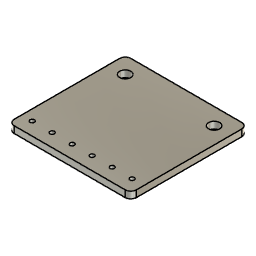
maze solevr part-1 v51 (Autodesk Fusion 360 archive; units mm, degrees)
design "ToF Distance Ranging Sensor"
Autodesk Fusion 360 part; units mm, degrees
sketch "Sketch1" plane through (0, 0, 0) normal (0, 0, 1) x (1, 0, 0)
  line L0 (21, 0.5) -> (21, 19.5)
  line L1 (-1, 19.5) -> (-1, 0.5)
  line L2 (20, 20.5) -> (0, 20.5)
  line L3 (0, -0.5) -> (20, -0.5)
  circle A0 centre (0.8946, 1.8577) radius 0.4
  circle A1 centre (4.4946, 1.8577) radius 0.4
  circle A2 centre (8.0946, 1.8577) radius 0.4
  circle A3 centre (11.6946, 1.8577) radius 0.4
  circle A4 centre (15.2946, 1.8577) radius 0.4
  circle A5 centre (18.8946, 1.8577) radius 0.4
  arc A6 (0, 20.5) -> (-1, 19.5) centre (0, 19.5) ccw
  arc A7 (21, 19.5) -> (20, 20.5) centre (20, 19.5) ccw
  arc A8 (-1, 0.5) -> (0, -0.5) centre (0, 0.5) ccw
  arc A9 (20, -0.5) -> (21, 0.5) centre (20, 0.5) ccw
  line L4 (-1, 20) -> (-1, 17.5)
  circle A10 centre (2, 17.5) radius 1
  circle A11 centre (18, 17.5) radius 1
  line L5 (17, 17.5) -> (18, 17.5)
  point P0 (20, 0)
  point P1 (0, 20)
  point P2 (9.789, 1.7034)
  point P3 (18.289, 1.7034)
  dimension "d1" = 20
  dimension "d2" = 20
  dimension "d30" = 0.8
  dimension "d33" = 18
  dimension "d34" = 0
  dimension "d35" = 1
  dimension "d36" = 2.5
  dimension "d37" = 3
  dimension "d38" = 2
  dimension "d39" = 2
  constraint tangent L2 A6
  constraint tangent L1 A6
  constraint tangent L2 A7
  constraint tangent L0 A7
  constraint equal A6 A7
  constraint tangent L1 A8
  constraint tangent L3 A8
  constraint equal A6 A8
  constraint tangent L0 A9
  constraint tangent L3 A9
  constraint equal A6 A9
  constraint parallel L1 L4
  constraint coincident A11.centre L5.end
  constraint coincident A11 L5.start
  measures "d1" distance of origin P0
  measures "d2" distance of origin P1
  measures "d30" diameter of A0
  measures "d35" radius of A6
  measures "d36" distance of L4.start L4.end
  measures "d37" distance of L4.end A10.centre
  measures "d38" diameter of A10
  measures "d39" diameter of A11
sketch "Sketch2" plane through (0, 0, 0) normal (0, 0, 1) x (1, 0, 0)
extrude "Extrude3" add sketch "Sketch1" along normal blind 1.21
extrude "Extrude2" [rolled back] along distance 1.21 taper angle 0

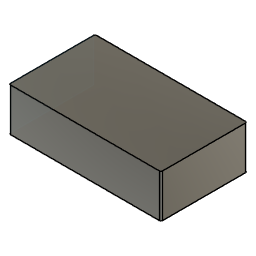
design "BATTERY"
Autodesk Fusion 360 part; units mm, degrees
sketch "Sketch1" plane through (0, 0, 0) normal (0, 0, 1) x (1, 0, 0)
  line L0 (0, 0) -> (53, 0)
  line L1 (53, 0) -> (53, 30)
  line L2 (53, 30) -> (0, 30)
  line L3 (0, 30) -> (0, 0)
  dimension "d1" = 53
  dimension "d2" = 30
  constraint horizontal L0
  constraint vertical L1
  constraint horizontal L2
  constraint vertical L3
  constraint coincident L0.start L3.end
  measures "d1" distance of L0.start L0.end
  measures "d2" distance of L0.start L2.end
extrude "Extrude1" add sketch "Sketch1" along normal blind 15
fillet "Fillet1" radius 0.5 1 edges at (0, 0, 7.5)
fillet "Fillet2" radius 0.5 3 edges at (53, 30, 7.5) (53, 0, 7.5) (0, 30, 7.5)
sketch "Sketch2" plane through (0, 0, 0) normal (-1, 0, 0) x (0, -1, 0)
  line L0 (-29.5, 15) -> (-29.5, 0)
  line L1 (-29.5, 0) -> (-0.5, 0)
  line L2 (-0.5, 0) -> (-0.5, 15)
  line L3 (-0.5, 15) -> (-29.5, 15)

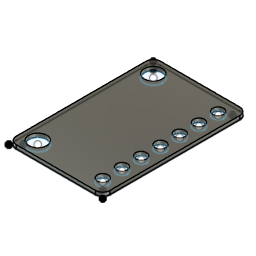
design "MAZE SOLVER WITH IMPELLER"
Autodesk Fusion 360 part; units mm, degrees
sketch "Sketch1" plane through (0, 0, 0) normal (0, 0, 1) x (1, 0, 0)
  line L0 (1, 0) -> (12, 0)
  line L1 (13, 1) -> (13, 19)
  line L2 (12, 20) -> (1, 20)
  line L3 (0, 19) -> (0, 1)
  circle A0 centre (2, 18) radius 1.25
  circle A1 centre (2, 2) radius 1.25
  arc A2 (1, 20) -> (0, 19) centre (1, 19) ccw
  arc A3 (0, 1) -> (1, 0) centre (1, 1) ccw
  arc A4 (13, 19) -> (12, 20) centre (12, 19) ccw
  arc A5 (12, 0) -> (13, 1) centre (12, 1) ccw
  circle A6 centre (11, 18) radius 0.75
  circle A7 centre (11, 15.3333) radius 0.75
  circle A8 centre (11, 12.6667) radius 0.75
  circle A9 centre (11, 10) radius 0.75
  circle A10 centre (11, 7.3333) radius 0.75
  circle A11 centre (11, 4.6667) radius 0.75
  circle A12 centre (11, 2) radius 0.75
  point P0 (13, 0)
  point P1 (0, 20)
  dimension "d1" = 13
  dimension "d2" = 20
  dimension "d3" = 2.5
  dimension "d4" = 2.5
  dimension "d5" = 1
  dimension "d6" = 1.5
  dimension "d9" = 0
  dimension "d10" = -16
  constraint horizontal L0
  constraint vertical L1
  constraint horizontal L2
  constraint vertical L3
  constraint coincident P1 L2
  constraint coincident P1 L3
  constraint tangent L2 A2
  constraint tangent L3 A2
  constraint coincident origin L3
  constraint coincident origin L0
  constraint tangent L3 A3
  constraint tangent L0 A3
  constraint equal A2 A3
  constraint tangent L2 A4
  constraint tangent L1 A4
  constraint equal A2 A4
  constraint coincident P0 L1
  constraint coincident P0 L0
  constraint tangent L1 A5
  constraint tangent L0 A5
  constraint equal A2 A5
  measures "d1" distance of origin P0
  measures "d2" distance of origin P1
  measures "d3" diameter of A0
  measures "d4" diameter of A1
  measures "d5" radius of A2
  measures "d6" diameter of A6
sketch "Sketch2" plane through (0, 0, 0) normal (0, 0, 1) x (1, 0, 0)
extrude "Extrude1" add sketch "Sketch1" along normal blind 0.5

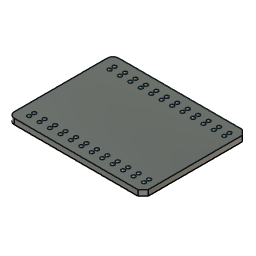
design "part-1 maze solver"
Autodesk Fusion 360 part; units mm, degrees
sketch "Sketch7" plane through (0, 0, 0) normal (0, 0, 1) x (1, 0, 0)
  line L0 (1.5, 0) -> (34.91, 0)
  line L1 (34.91, 28.14) -> (1.5, 28.14)
  line L2 (0, 26.64) -> (0, 1.5)
  line L3 (34.91, 28.14) -> (36.28, 26.77)
  line L4 (34.91, 0) -> (36.28, 1.37)
  arc A0 (1.5, 28.14) -> (0, 26.64) centre (1.5, 26.64) ccw
  arc A1 (0, 1.5) -> (1.5, 0) centre (1.5, 1.5) ccw
  circle A2 centre (3, 25.6) radius 0.5
  circle A3 centre (3, 24.23) radius 0.5
  circle A4 centre (3, 3.91) radius 0.5
  circle A5 centre (3, 2.54) radius 0.5
  circle A6 centre (5.8182, 25.6) radius 0.5
  circle A7 centre (5.8182, 24.23) radius 0.5
  circle A8 centre (8.6364, 25.6) radius 0.5
  circle A9 centre (8.6364, 24.23) radius 0.5
  circle A10 centre (11.4545, 25.6) radius 0.5
  circle A11 centre (11.4545, 24.23) radius 0.5
  circle A12 centre (14.2727, 24.23) radius 0.5
  circle A13 centre (17.0909, 25.6) radius 0.5
  circle A14 centre (17.0909, 24.23) radius 0.5
  circle A15 centre (19.9091, 25.6) radius 0.5
  circle A16 centre (19.9091, 24.23) radius 0.5
  circle A17 centre (22.7273, 25.6) radius 0.5
  circle A18 centre (22.7273, 24.23) radius 0.5
  circle A19 centre (25.5455, 25.6) radius 0.5
  circle A20 centre (25.5455, 24.23) radius 0.5
  circle A21 centre (28.3636, 25.6) radius 0.5
  circle A22 centre (28.3636, 24.23) radius 0.5
  circle A23 centre (31.1818, 25.6) radius 0.5
  circle A24 centre (31.1818, 24.23) radius 0.5
  circle A25 centre (34, 25.6) radius 0.5
  circle A26 centre (34, 24.23) radius 0.5
  circle A27 centre (5.8182, 3.91) radius 0.5
  circle A28 centre (5.8182, 2.54) radius 0.5
  circle A29 centre (8.6364, 3.91) radius 0.5
  circle A30 centre (8.6364, 2.54) radius 0.5
  circle A31 centre (11.4545, 3.91) radius 0.5
  circle A32 centre (11.4545, 2.54) radius 0.5
  circle A33 centre (14.2727, 3.91) radius 0.5
  circle A34 centre (14.2727, 2.54) radius 0.5
  circle A35 centre (17.0909, 3.91) radius 0.5
  circle A36 centre (17.0909, 2.54) radius 0.5
  circle A37 centre (19.9091, 3.91) radius 0.5
  circle A38 centre (19.9091, 2.54) radius 0.5
  circle A39 centre (22.7273, 3.91) radius 0.5
  circle A40 centre (22.7273, 2.54) radius 0.5
  circle A41 centre (25.5455, 3.91) radius 0.5
  circle A42 centre (25.5455, 2.54) radius 0.5
  circle A43 centre (28.3636, 3.91) radius 0.5
  circle A44 centre (28.3636, 2.54) radius 0.5
  circle A45 centre (31.1818, 3.91) radius 0.5
  circle A46 centre (31.1818, 2.54) radius 0.5
  circle A47 centre (34, 3.91) radius 0.5
  circle A48 centre (34, 2.54) radius 0.5
  line L5 (3, 4.41) -> (3, 3.91)
  line L6 (30.6818, 3.91) -> (31.6818, 3.91)
  line L7 (33.5, 3.91) -> (34.5, 3.91)
  line L8 (30.6845, 2.4881) -> (31.6789, 2.4862)
  line L9 (33.5033, 2.4828) -> (34.4965, 2.4809)
  circle A49 centre (14.2727, 25.6) radius 0.5
  line L10 (36.28, 26.77) -> (36.28, 1.37)
  point P0 (0, 28.14)
  dimension "d40" = 28.14
  dimension "d45" = 1.5
  dimension "d49" = 1.37
  dimension "d50" = 1
  dimension "d51" = 1
  dimension "d52" = 1
  dimension "d53" = 1
  dimension "d56" = 31
  dimension "d57" = 0
  dimension "d60" = 31
  dimension "d61" = 0
  dimension "d62" = 1
  constraint horizontal L0
  constraint horizontal L1
  constraint vertical L2
  constraint coincident P0 L1
  constraint coincident P0 L2
  constraint tangent L1 A0
  constraint tangent L2 A0
  constraint coincident origin L2
  constraint coincident origin L0
  constraint tangent L2 A1
  constraint tangent L0 A1
  constraint equal A0 A1
  constraint coincident A4.centre L5.end
  constraint coincident A4 L5.start
  constraint coincident A46 L8.start
  constraint coincident A45 L6.start
  constraint coincident A45 L6.end
  constraint coincident A47 L7.start
  constraint collinear L6 L7
  constraint coincident A46 L8.end
  constraint coincident A48 L9.start
  constraint collinear L8 L9
  constraint coincident A48 L9.end
  constraint coincident A47 L7.end
  constraint vertical L10
  measures "d40" distance of origin P0
  measures "d45" radius of A0
  measures "d49" distance of A4.centre A5.centre
  measures "d50" diameter of A2
  measures "d51" diameter of A3
  measures "d52" diameter of A4
  measures "d53" diameter of A5
  measures "d62" diameter of A49
extrude "Extrude4" add sketch "Sketch7" along normal blind 1.5
sketch "Sketch8" plane through (0, 0, 0) normal (0, 0, -1) x (1, 0, 0)
  circle A0 centre (34, -3.91) radius 0.5
  circle A1 centre (25.5455, -2.54) radius 0.5
  circle A2 centre (11.4545, -3.91) radius 0.5
  circle A3 centre (14.2727, -3.91) radius 0.5
  circle A4 centre (19.9091, -25.6) radius 0.5
  circle A5 centre (17.0909, -24.23) radius 0.5
  circle A6 centre (5.8182, -3.91) radius 0.5
  circle A7 centre (3, -3.91) radius 0.5
  circle A8 centre (11.4545, -24.23) radius 0.5
  circle A9 centre (34, -2.54) radius 0.5
  circle A10 centre (8.6364, -24.23) radius 0.5
  circle A11 centre (25.5455, -24.23) radius 0.5
  circle A12 centre (28.3636, -24.23) radius 0.5
  circle A13 centre (34, -25.6) radius 0.5
  circle A14 centre (8.6364, -2.54) radius 0.5
  circle A15 centre (22.7273, -25.6) radius 0.5
  circle A16 centre (28.3636, -25.6) radius 0.5
  circle A17 centre (3, -24.23) radius 0.5
  circle A18 centre (25.5455, -3.91) radius 0.5
  circle A19 centre (17.0909, -2.54) radius 0.5
  circle A20 centre (3, -25.6) radius 0.5
  circle A21 centre (14.2727, -25.6) radius 0.5
  circle A22 centre (5.8182, -24.23) radius 0.5
  circle A23 centre (19.9091, -3.91) radius 0.5
  circle A24 centre (22.7273, -2.54) radius 0.5
  circle A25 centre (28.3636, -2.54) radius 0.5
  circle A26 centre (5.8182, -2.54) radius 0.5
  circle A27 centre (28.3636, -3.91) radius 0.5
  circle A28 centre (14.2727, -24.23) radius 0.5
  circle A29 centre (5.8182, -25.6) radius 0.5
  circle A30 centre (34, -24.23) radius 0.5
  circle A31 centre (19.9091, -24.23) radius 0.5
  circle A32 centre (14.2727, -2.54) radius 0.5
  circle A33 centre (31.1818, -25.6) radius 0.5
  circle A34 centre (19.9091, -2.54) radius 0.5
  circle A35 centre (25.5455, -25.6) radius 0.5
  circle A36 centre (11.4545, -25.6) radius 0.5
  circle A37 centre (31.1818, -3.91) radius 0.5
  circle A38 centre (8.6364, -3.91) radius 0.5
  circle A39 centre (17.0909, -25.6) radius 0.5
  circle A40 centre (3, -2.54) radius 0.5
  circle A41 centre (17.0909, -3.91) radius 0.5
  circle A42 centre (8.6364, -25.6) radius 0.5
  circle A43 centre (31.1818, -2.54) radius 0.5
  circle A44 centre (31.1818, -24.23) radius 0.5
  circle A45 centre (11.4545, -2.54) radius 0.5
  circle A46 centre (22.7273, -3.91) radius 0.5
  circle A47 centre (22.7273, -24.23) radius 0.5
  line L0 (1.5, -28.14) -> (34.91, -28.14)
  line L1 (34.91, -28.14) -> (36.28, -26.77)
  line L2 (36.28, -26.77) -> (36.28, -1.37)
  line L3 (36.28, -1.37) -> (34.91, 0)
  line L4 (34.91, 0) -> (1.5, 0)
  arc A48 (1.5, 0) -> (0, -1.5) centre (1.5, -1.5) ccw
  line L5 (0, -1.5) -> (0, -26.64)
  arc A49 (0, -26.64) -> (1.5, -28.14) centre (1.5, -26.64) ccw
  line L6 (0.4393, -2.2046) -> (2.0598, -2.2046)
  line L7 (2.0598, -2.2046) -> (2.0598, -4.4608)
  line L8 (2.0598, -4.4608) -> (0.4393, -4.4608)
  line L9 (0.4393, -4.4608) -> (0.4393, -2.2046)
  line L10 (0.4393, -24.1927) -> (2.0598, -24.1927)
  line L11 (2.0598, -24.1927) -> (2.0598, -26.4526)
  line L12 (2.0598, -26.4526) -> (0.4393, -26.4526)
  line L13 (0.4393, -26.4526) -> (0.4393, -24.1927)
  constraint horizontal L6
  constraint vertical L7
  constraint horizontal L8
  constraint vertical L9
  constraint horizontal L10
  constraint vertical L11
  constraint horizontal L12
  constraint vertical L13
extrude "Extrude5" add sketch "Sketch8" along normal blind 0.5 contours L6 L7 L8 L9 | L10 L11 L12 L13
sketch "Sketch9" plane through (0, 0, 0) normal (0, 0, -1) x (1, 0, 0)
  line L0 (0.4393, -26.4526) -> (0.4393, -24.1927)
  line L1 (0.4393, -24.1927) -> (2.0598, -24.1927)
  line L2 (2.0598, -24.1927) -> (2.0598, -26.4526)
  line L3 (2.0598, -26.4526) -> (0.4393, -26.4526)
  line L4 (0.4393, -4.4608) -> (0.4393, -2.2046)
  line L5 (0.4393, -2.2046) -> (2.0598, -2.2046)
  line L6 (2.0598, -2.2046) -> (2.0598, -4.4608)
  line L7 (2.0598, -4.4608) -> (0.4393, -4.4608)
  circle A0 centre (34, -3.91) radius 0.5
  circle A1 centre (25.5455, -2.54) radius 0.5
  circle A2 centre (11.4545, -3.91) radius 0.5
  circle A3 centre (14.2727, -3.91) radius 0.5
  circle A4 centre (19.9091, -25.6) radius 0.5
  circle A5 centre (17.0909, -24.23) radius 0.5
  circle A6 centre (5.8182, -3.91) radius 0.5
  circle A7 centre (3, -3.91) radius 0.5
  circle A8 centre (11.4545, -24.23) radius 0.5
  circle A9 centre (34, -2.54) radius 0.5
  circle A10 centre (8.6364, -24.23) radius 0.5
  circle A11 centre (25.5455, -24.23) radius 0.5
  circle A12 centre (28.3636, -24.23) radius 0.5
  circle A13 centre (34, -25.6) radius 0.5
  circle A14 centre (8.6364, -2.54) radius 0.5
  circle A15 centre (22.7273, -25.6) radius 0.5
  circle A16 centre (28.3636, -25.6) radius 0.5
  circle A17 centre (3, -24.23) radius 0.5
  circle A18 centre (25.5455, -3.91) radius 0.5
  circle A19 centre (17.0909, -2.54) radius 0.5
  circle A20 centre (3, -25.6) radius 0.5
  circle A21 centre (14.2727, -25.6) radius 0.5
  circle A22 centre (5.8182, -24.23) radius 0.5
  circle A23 centre (19.9091, -3.91) radius 0.5
  circle A24 centre (22.7273, -2.54) radius 0.5
  circle A25 centre (28.3636, -2.54) radius 0.5
  circle A26 centre (5.8182, -2.54) radius 0.5
  circle A27 centre (28.3636, -3.91) radius 0.5
  circle A28 centre (14.2727, -24.23) radius 0.5
  circle A29 centre (5.8182, -25.6) radius 0.5
  circle A30 centre (34, -24.23) radius 0.5
  circle A31 centre (19.9091, -24.23) radius 0.5
  circle A32 centre (14.2727, -2.54) radius 0.5
  circle A33 centre (31.1818, -25.6) radius 0.5
  circle A34 centre (19.9091, -2.54) radius 0.5
  circle A35 centre (25.5455, -25.6) radius 0.5
  circle A36 centre (11.4545, -25.6) radius 0.5
  circle A37 centre (31.1818, -3.91) radius 0.5
  circle A38 centre (8.6364, -3.91) radius 0.5
  circle A39 centre (17.0909, -25.6) radius 0.5
  circle A40 centre (3, -2.54) radius 0.5
  circle A41 centre (17.0909, -3.91) radius 0.5
  circle A42 centre (8.6364, -25.6) radius 0.5
  circle A43 centre (31.1818, -2.54) radius 0.5
  circle A44 centre (31.1818, -24.23) radius 0.5
  circle A45 centre (11.4545, -2.54) radius 0.5
  circle A46 centre (22.7273, -3.91) radius 0.5
  circle A47 centre (22.7273, -24.23) radius 0.5
  line L8 (1.5, -28.14) -> (34.91, -28.14)
  line L9 (34.91, -28.14) -> (36.28, -26.77)
  line L10 (36.28, -26.77) -> (36.28, -1.37)
  line L11 (36.28, -1.37) -> (34.91, 0)
  line L12 (34.91, 0) -> (1.5, 0)
  arc A48 (1.5, 0) -> (0, -1.5) centre (1.5, -1.5) ccw
  line L13 (0, -1.5) -> (0, -26.64)
  arc A49 (0, -26.64) -> (1.5, -28.14) centre (1.5, -26.64) ccw
sketch "Sketch10" plane through (0, 0, 1.5) normal (0, 0, 1) x (-1, 0, 0)
  circle A0 centre (-34, -3.91) radius 0.5
  circle A1 centre (-25.5455, -2.54) radius 0.5
  circle A2 centre (-11.4545, -3.91) radius 0.5
  circle A3 centre (-14.2727, -3.91) radius 0.5
  circle A4 centre (-19.9091, -25.6) radius 0.5
  circle A5 centre (-17.0909, -24.23) radius 0.5
  circle A6 centre (-5.8182, -3.91) radius 0.5
  circle A7 centre (-3, -3.91) radius 0.5
  circle A8 centre (-11.4545, -24.23) radius 0.5
  circle A9 centre (-34, -2.54) radius 0.5
  circle A10 centre (-8.6364, -24.23) radius 0.5
  circle A11 centre (-25.5455, -24.23) radius 0.5
  circle A12 centre (-28.3636, -24.23) radius 0.5
  circle A13 centre (-34, -25.6) radius 0.5
  circle A14 centre (-8.6364, -2.54) radius 0.5
  circle A15 centre (-22.7273, -25.6) radius 0.5
  circle A16 centre (-28.3636, -25.6) radius 0.5
  circle A17 centre (-3, -24.23) radius 0.5
  circle A18 centre (-25.5455, -3.91) radius 0.5
  circle A19 centre (-17.0909, -2.54) radius 0.5
  circle A20 centre (-3, -25.6) radius 0.5
  circle A21 centre (-14.2727, -25.6) radius 0.5
  circle A22 centre (-5.8182, -24.23) radius 0.5
  circle A23 centre (-19.9091, -3.91) radius 0.5
  circle A24 centre (-22.7273, -2.54) radius 0.5
  circle A25 centre (-28.3636, -2.54) radius 0.5
  circle A26 centre (-5.8182, -2.54) radius 0.5
  circle A27 centre (-28.3636, -3.91) radius 0.5
  circle A28 centre (-14.2727, -24.23) radius 0.5
  circle A29 centre (-5.8182, -25.6) radius 0.5
  circle A30 centre (-34, -24.23) radius 0.5
  circle A31 centre (-19.9091, -24.23) radius 0.5
  circle A32 centre (-14.2727, -2.54) radius 0.5
  circle A33 centre (-31.1818, -25.6) radius 0.5
  circle A34 centre (-19.9091, -2.54) radius 0.5
  circle A35 centre (-25.5455, -25.6) radius 0.5
  circle A36 centre (-11.4545, -25.6) radius 0.5
  circle A37 centre (-31.1818, -3.91) radius 0.5
  circle A38 centre (-8.6364, -3.91) radius 0.5
  circle A39 centre (-17.0909, -25.6) radius 0.5
  circle A40 centre (-3, -2.54) radius 0.5
  circle A41 centre (-17.0909, -3.91) radius 0.5
  circle A42 centre (-8.6364, -25.6) radius 0.5
  circle A43 centre (-31.1818, -2.54) radius 0.5
  circle A44 centre (-31.1818, -24.23) radius 0.5
  circle A45 centre (-11.4545, -2.54) radius 0.5
  circle A46 centre (-22.7273, -3.91) radius 0.5
  circle A47 centre (-22.7273, -24.23) radius 0.5
  line L0 (-34.91, -28.14) -> (-1.5, -28.14)
  arc A48 (-1.5, -28.14) -> (0, -26.64) centre (-1.5, -26.64) ccw
  line L1 (0, -26.64) -> (0, -1.5)
  arc A49 (0, -1.5) -> (-1.5, 0) centre (-1.5, -1.5) ccw
  line L2 (-1.5, 0) -> (-34.91, 0)
  line L3 (-34.91, 0) -> (-36.28, -1.37)
  line L4 (-36.28, -1.37) -> (-36.28, -26.77)
  line L5 (-36.28, -26.77) -> (-34.91, -28.14)

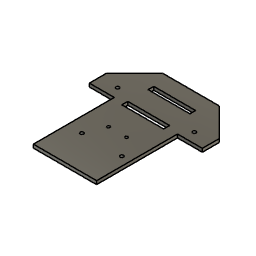
design "top layer"
Autodesk Fusion 360 part; units mm, degrees
sketch "Sketch11" plane through (0, 0, 0) normal (0, 0, 1) x (1, 0, 0)
  line L0 (0, 0) -> (56, 0)
  line L1 (56, 0) -> (56, 70)
  line L2 (0, 70) -> (0, 0)
  line L3 (0, 70) -> (-22, 70)
  line L4 (-22, 70) -> (-22, 85)
  line L5 (56, 70) -> (78, 70)
  line L6 (78, 70) -> (78, 85)
  line L7 (78, 85) -> (53.0002, 109.9998)
  line L8 (-22, 85) -> (2.9998, 109.9998)
  line L9 (-22, 85) -> (13.355, 85) construction
  line L10 (2.9998, 109.9998) -> (53.0002, 109.9998)
  dimension "d57" = 56
  dimension "d58" = 70
  dimension "d59" = 22
  dimension "d60" = 15
  dimension "d61" = 22
  dimension "d62" = 135
  dimension "d63" = 35.355
  dimension "d64" = 45
  dimension "d65" = 35.355
  constraint horizontal L0
  constraint vertical L1
  constraint vertical L2
  constraint coincident L0.start L2.end
  constraint perpendicular L2 L3
  constraint vertical L4
  constraint perpendicular L1 L5
  constraint perpendicular L5 L6
  constraint horizontal L9
  constraint horizontal L10
  measures "d57" distance of L0.start L0.end
  measures "d58" distance of L0.start L2.start
  measures "d59" distance of L2.start L3.end
  measures "d60" distance of L3.end L4.end
  measures "d61" distance of L1.end L5.end
  measures "d62" angle of L6 L7
  measures "d63" distance of L6.end L7.end
  measures "d64" angle of L8 L9
  measures "d65" distance of L4.end L8.end
extrude "Extrude14" add sketch "Sketch11" along normal blind 3
extrude "Extrude15" add 1 faces at (18.6667, 0, 1) along direction (0, -1, 0) blind 1.6
sketch "Sketch12" plane through (0, 0, 3) normal (0, 0, 1) x (-1, 0, 0)
  line L0 (0, -70) -> (0, 1.6)
  line L1 (0, 1.6) -> (-56, 1.6)
  line L2 (-56, 1.6) -> (-56, -70)
  line L3 (-56, -70) -> (-78, -70)
  line L4 (-78, -70) -> (-78, -85)
  line L5 (-78, -85) -> (-53.0002, -109.9998)
  line L6 (-53.0002, -109.9998) -> (-2.9998, -109.9998)
  line L7 (-2.9998, -109.9998) -> (22, -85)
  line L8 (22, -85) -> (22, -70)
  line L9 (22, -70) -> (0, -70)
  circle A0 centre (6, -79) radius 1.5
  circle A1 centre (-62, -79) radius 1.5
  line L10 (0, 1.6) -> (-28, 1.6)
  circle A2 centre (-13, -28.42) radius 1.5
  circle A3 centre (-48.387, -28.42) radius 1.5
  dimension "d72" = 3
  dimension "d75" = 3
  dimension "d78" = 35.387
  dimension "d79" = 3
  dimension "d80" = 3
  constraint coincident L0.end L1.start
  constraint midpoint L1 L10.end
  measures "d72" diameter of A0
  measures "d75" diameter of A1
  measures "d78" distance of A2.centre A3.centre
  measures "d79" diameter of A2
  measures "d80" diameter of A3
extrude "Extrude16" cut sketch "Sketch12" against normal blind 195 contours A0 | A1 | A2 | A3
sketch "Sketch13" plane through (0, 0, 3) normal (0, 0, 1) x (-1, 0, 0)
  circle A0 centre (-48.387, -28.42) radius 1.5
  circle A1 centre (6, -79) radius 1.5
  circle A2 centre (-13, -28.42) radius 1.5
  circle A3 centre (-62, -79) radius 1.5
  line L0 (0, -70) -> (0, 1.6)
  line L1 (0, 1.6) -> (-56, 1.6)
  line L2 (-56, 1.6) -> (-56, -70)
  line L3 (-56, -70) -> (-78, -70)
  line L4 (-78, -70) -> (-78, -85)
  line L5 (-78, -85) -> (-53.0002, -109.9998)
  line L6 (-53.0002, -109.9998) -> (-2.9998, -109.9998)
  line L7 (-2.9998, -109.9998) -> (22, -85)
  line L8 (22, -85) -> (22, -70)
  line L9 (22, -70) -> (0, -70)
  line L10 (0, -70) -> (0, -45)
  line L11 (0, -45) -> (-20, -45)
  circle A4 centre (-20, -45) radius 1.25
  line L12 (-56, -70) -> (-56, -45)
  line L13 (-56, -45) -> (-36, -45)
  circle A5 centre (-36, -45) radius 1.25
  dimension "d83" = 25
  dimension "d84" = 20
  dimension "d85" = 2.5
  dimension "d86" = 25
  dimension "d87" = 20
  dimension "d88" = 2.5
  constraint coincident L0.start L9.end
  constraint perpendicular L9 L10
  constraint perpendicular L10 L11
  constraint coincident L11.end A4.centre
  constraint coincident L2.end L3.start
  constraint perpendicular L3 L12
  constraint perpendicular L12 L13
  constraint coincident L13.end A5.centre
  measures "d83" distance of L0.start L10.end
  measures "d84" distance of L10.end L11.end
  measures "d85" diameter of A4
  measures "d86" distance of L2.end L12.end
  measures "d87" distance of L12.end L13.end
  measures "d88" diameter of A5
extrude "Extrude17" cut sketch "Sketch13" against normal blind 48 contours A4 | A5
sketch "Sketch14" plane through (0, 0, 3) normal (0, 0, 1) x (-1, 0, 0)
  circle A0 centre (-20, -45) radius 1.25
  circle A1 centre (-36, -45) radius 1.25
  circle A2 centre (-48.387, -28.42) radius 1.5
  circle A3 centre (6, -79) radius 1.5
  circle A4 centre (-13, -28.42) radius 1.5
  circle A5 centre (-62, -79) radius 1.5
  line L0 (0, -70) -> (0, 1.6)
  line L1 (0, 1.6) -> (-56, 1.6)
  line L2 (-56, 1.6) -> (-56, -70)
  line L3 (-56, -70) -> (-78, -70)
  line L4 (-78, -70) -> (-78, -85)
  line L5 (-78, -85) -> (-53.0002, -109.9998)
  line L6 (-53.0002, -109.9998) -> (-2.9998, -109.9998)
  line L7 (-2.9998, -109.9998) -> (22, -85)
  line L8 (22, -85) -> (22, -70)
  line L9 (22, -70) -> (0, -70)
  line L10 (0, -70) -> (-9, -70)
  line L11 (-9, -70) -> (-9, -73)
  line L12 (-9, -73) -> (-46, -73)
  line L13 (-46, -73) -> (-46, -67.745)
  line L14 (-46, -67.745) -> (-9, -67.745)
  line L15 (-9, -70) -> (-9, -67.745)
  line L16 (-9, -73) -> (-9, -96)
  line L17 (-9, -96) -> (-46, -96)
  line L18 (-46, -96) -> (-46, -92)
  line L19 (-46, -92) -> (-9, -92)
  line L20 (-9, -96) -> (-9, -92)
  dimension "d91" = 9
  dimension "d92" = 37
  dimension "d93" = 5.255
  dimension "d94" = 23
  dimension "d95" = 37
  dimension "d96" = 4
  constraint coincident L0.start L9.end
  constraint perpendicular L0 L10
  constraint perpendicular L10 L11
  constraint perpendicular L0 L12
  constraint perpendicular L12 L13
  constraint perpendicular L13 L14
  constraint perpendicular L14 L15
  constraint perpendicular L12 L16
  constraint perpendicular L16 L17
  constraint perpendicular L17 L18
  constraint coincident L16 L19.end
  constraint perpendicular L16 L19
  measures "d91" distance of L0.start L10.end
  measures "d92" distance of L11.end L12.end
  measures "d93" distance of L12.end L13.end
  measures "d94" distance of L11.end L16.end
  measures "d95" distance of L16.end L17.end
  measures "d96" distance of L17.end L18.end
extrude "Extrude18" cut sketch "Sketch14" against normal blind 73 contours L11 L12 L13 L14 L15 | L16 L17 L18 L19 L20
extrude "Extrude19" cut 1 faces at (33.6667, 92, 1) along direction (0, -1, 0) blind 1
sketch "Sketch15" plane through (0, 0, 3) normal (0, 0, 1) x (-1, 0, 0)
  line L0 (0, -70) -> (6, -70)
  constraint horizontal L0
sketch "Sketch16" plane through (0, 0, 3) normal (0, 0, 1) x (-1, 0, 0)
  line L0 (0, -70) -> (0, 1.6)
  line L1 (0, 1.6) -> (-56, 1.6)
  line L2 (-56, 1.6) -> (-56, -70)
  line L3 (-56, -70) -> (-78, -70)
  line L4 (-78, -70) -> (-78, -85)
  line L5 (-78, -85) -> (-53.0002, -109.9998)
  line L6 (-53.0002, -109.9998) -> (-2.9998, -109.9998)
  line L7 (-2.9998, -109.9998) -> (22, -85)
  line L8 (22, -85) -> (22, -70)
  line L9 (22, -70) -> (0, -70)
  circle A0 centre (-62, -79) radius 1.5
  circle A1 centre (-13, -28.42) radius 1.5
  circle A2 centre (6, -79) radius 1.5
  circle A3 centre (-48.387, -28.42) radius 1.5
  circle A4 centre (-36, -45) radius 1.25
  circle A5 centre (-20, -45) radius 1.25
  line L10 (-46, -96) -> (-46, -91)
  line L11 (-46, -91) -> (-9, -91)
  line L12 (-9, -91) -> (-9, -96)
  line L13 (-9, -96) -> (-46, -96)
  line L14 (-46, -67.745) -> (-9, -67.745)
  line L15 (-9, -67.745) -> (-9, -73)
  line L16 (-9, -73) -> (-46, -73)
  line L17 (-46, -73) -> (-46, -67.745)

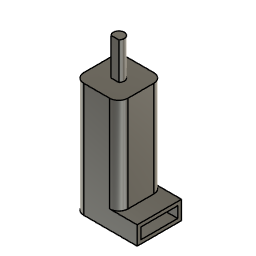
design "rough sketch of n20 motor"
Autodesk Fusion 360 part; units mm, degrees
sketch "Sketch1" plane through (0, 0, 0) normal (0, 0, 1) x (1, 0, 0)
  line L0 (0, 0) -> (12, 0)
  line L1 (12, 0) -> (12, 12)
  line L2 (12, 12) -> (0, 12)
  line L3 (0, 12) -> (0, 0)
  dimension "d1" = 12
  dimension "d2" = 12
  constraint horizontal L0
  constraint vertical L1
  constraint horizontal L2
  constraint vertical L3
  constraint coincident L0.start L3.end
  measures "d1" distance of L0.start L0.end
  measures "d2" distance of L0.start L2.end
extrude "Extrude1" add sketch "Sketch1" along normal blind 31
sketch "Sketch2" plane through (12, 0, 0) normal (1, 0, 0) x (0, 1, 0)
  line L0 (0, 0) -> (12, 0)
  line L1 (12, 0) -> (12, 31)
  line L2 (12, 31) -> (0, 31)
  line L3 (0, 31) -> (0, 0)
  line L4 (0, 0) -> (0, 5)
  line L5 (0, 5) -> (12, 5)
  line L6 (12, 5) -> (12, 0)
  line L7 (0, 0) -> (12, 0)
  dimension "d5" = 5
  constraint coincident L0.start L3.end
  constraint perpendicular L0 L4
  constraint coincident L1 L5.end
  constraint perpendicular L1 L5
  constraint coincident L0.end L1.start
  measures "d5" distance of L0.start L4.end
extrude "Extrude2" add sketch "Sketch2" along normal blind 5 contours L0 L1 L3 L4 L5 L6 L7
sketch "Sketch3" plane through (17, 0, 0) normal (1, 0, 0) x (0, 1, 0)
  line L0 (0, 5) -> (0, 0)
  line L1 (0, 0) -> (12, 0)
  line L2 (12, 0) -> (12, 5)
  line L3 (12, 5) -> (0, 5)
  line L4 (1, 4) -> (11, 4)
  line L5 (11, 4) -> (11, 1)
  line L6 (11, 1) -> (1, 1)
  line L7 (1, 1) -> (1, 4)
  constraint horizontal L4
  constraint vertical L5
  constraint horizontal L6
  constraint vertical L7
extrude "Extrude3" cut sketch "Sketch3" against normal blind 4 contours L4 L5 L6 L7
fillet "Fillet1" radius 2.5 4 edges at (12, 0, 18) (0, 0, 15.5) (12, 12, 18) (0, 12, 15.5)
sketch "Sketch4" plane through (0, 0, 31) normal (0, 0, 1) x (-1, 0, 0)
  arc A0 (-2.5, -12) -> (0, -9.5) centre (-2.5, -9.5) ccw
  line L0 (0, -9.5) -> (0, -2.5)
  arc A1 (0, -2.5) -> (-2.5, 0) centre (-2.5, -2.5) ccw
  line L1 (-2.5, 0) -> (-9.5, 0)
  arc A2 (-9.5, 0) -> (-12, -2.5) centre (-9.5, -2.5) ccw
  line L2 (-12, -2.5) -> (-12, -9.5)
  arc A3 (-12, -9.5) -> (-9.5, -12) centre (-9.5, -9.5) ccw
  line L3 (-9.5, -12) -> (-2.5, -12)
  line L4 (-7.0767, -4.9556) -> (-4.9233, -4.9556)
  arc A4 (-7.0767, -4.9556) -> (-4.9233, -4.9556) centre (-6, -6) ccw
  dimension "d12" = 3
  constraint horizontal L4
  measures "d12" diameter of A4
extrude "Extrude4" add sketch "Sketch4" along normal blind 10 contours L4 A4
